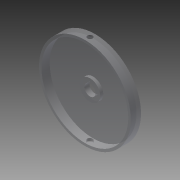
# Autodesk Inventor part: rotor
Saved by Autodesk Inventor 2014 (Build 180170000, 170)
## iProperties
Created: 2015-03-19
Part Number: rotor
Material: PMMA Plastic
Document SubType Name: Modeling
Designer: MSI
Density: 1 g/cm^3
Appearance: Polycarbonate - Clear
Author: MSI
Autodesk Inventor part; units mm, degrees
ref_plane "YZ Plane" through (0, 0, 0) normal (1, 0, 0) x (0, 1, 0)
ref_plane "XZ Plane" through (0, 0, 0) normal (0, 1, 0) x (-1, 0, 0)
sketch "Sketch1" plane through (0, 0, 0) normal (0, 1, 0) x (-1, 0, 0)
  circle A0 centre (0, 0) radius 45
  dimension "d0" = 90
  constraints: 1 centre point, 1 coincident
  measures "d0" diameter of A0
extrude "Extrusion1" add sketch "Sketch1" along normal blind 10
sketch "Sketch2" plane through (0, 0, 0) normal (0, -1, 0) x (1, 0, 0)
  circle A0 centre (0, 0) radius 45 projected
  circle A1 centre (0, 0) radius 42.5
  dimension "d3" = 85
  constraints: 1 centre point, 1 coincident
  measures "d3" diameter of A1
extrude "Extrusion2" cut sketch "Sketch2" against normal blind 5 contours A1
sketch "Sketch3" plane through (0, 5, 0) normal (0, -1, 0) x (1, 0, 0)
  circle A0 centre (0, 0) radius 42.5 projected
  circle A1 centre (0, 0) radius 10
  dimension "d6" = 20
  constraints: 1 centre point, 1 coincident
  measures "d6" diameter of A1
extrude "Extrusion3" cut sketch "Sketch3" against normal blind 3
sketch "Sketch4" plane through (0, 5, 0) normal (0, -1, 0) x (1, 0, 0)
  circle A0 centre (0, 0) radius 10 projected
  constraints: 1 coincident
hole "Hole1" at (0, 5, 0) direction (0, 1, 0) diameter 11 end through all
ref_plane "Work Plane1" through (0, 0, 45) normal (0, 0, 1) x (1, 0, 0)
sketch "Sketch5" plane through (0, 0, 45) normal (0, 0, 1) x (1, 0, 0)
  point P0 (0, 0)
  point P1 (0, 5)
  dimension "d17" = 5
  constraints: 1 vertical alignment
  measures "d17" distance of point (0, 0) point (0, 5)
ref_plane "Work Plane2" through (0, 0, -45) normal (0, 0, 1) x (1, 0, 0)
sketch "Sketch6" plane through (0, 0, -45) normal (0, 0, 1) x (1, 0, 0)
  point P0 (0, 0)
  point P1 (0, 5)
  dimension "d19" = 5
  constraints: 1 vertical alignment
  measures "d19" distance of point (0, 0) point (0, 5)
hole "Hole2" at (0, 5, 45) direction (0, 0, -1) diameter 5 depth 8 tip angle 118
hole "Hole3" at (0, 5, -45) direction (0, 0, 1) diameter 5 depth 8 tip angle 118
body "Solid1"
